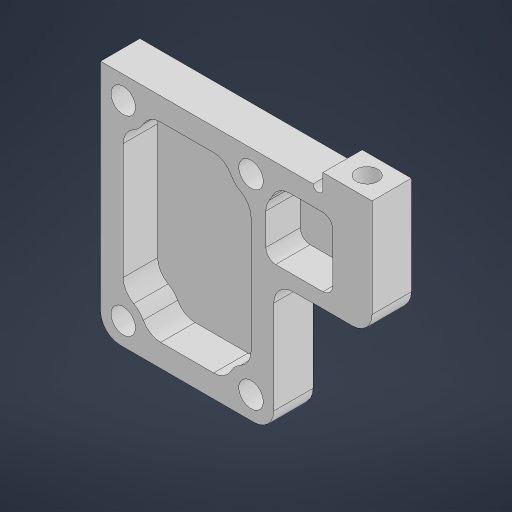
# Autodesk Inventor part: SolenoidMount
Saved by Autodesk Inventor 2024.2 (Build 282272000, 272)
## iProperties
Created: 2023-12-22
Part Number: SolenoidMount
Material: 一般
Document SubType Name: Modeling
Designer: Hanaoka
Density: 1 g/cm^3
Appearance: 既定
Author: Hanaoka
Autodesk Inventor part; units mm, degrees
ref_plane "YZ Plane" through (0, 0, 0) normal (1, 0, 0) x (0, 1, 0)
ref_plane "XZ Plane" through (0, 0, 0) normal (0, 1, 0) x (-1, 0, 0)
ref_plane "XY Plane" through (0, 0, 0) normal (0, 0, 1) x (1, 0, 0)
ref_plane "作業平面1" through (0, 0, 0.15) normal (0, 0, 1) x (1, 0, 0)
sketch "スケッチ1" plane through (0, 0, 0.15) normal (0, 0, 1) x (1, 0, 0)
  line L0 (0, -24) -> (-27.3, -24) projected
  line L1 (-3.7, -24) -> (-3.7, -10.5)
  line L2 (-3.7, -10.5) -> (4.3, -10.5)
  line L3 (6.3, -8.5) -> (6.3, 1.5)
  line L4 (6.3, 1.5) -> (1.3, 1.5)
  line L5 (-27.3, 0) -> (0, 0) projected
  line L6 (1.3, 1.5) -> (1.3, 0)
  circle A0 centre (-6, -21.7) radius 1.25 projected
  circle A1 centre (-19, -21.7) radius 1.25 projected
  circle A2 centre (-6, -21.7) radius 2.3 construction
  circle A3 centre (-19, -21.7) radius 2.3 construction
  line L7 (1.3, 0) -> (0, 0)
  line L8 (-21.3, -24) -> (-21.3, 0)
  circle A4 centre (-6, -2.3) radius 1.25 projected
  circle A5 centre (-19, -2.3) radius 1.25 projected
  line L9 (1.3, 0) -> (0.8, 0)
  arc A6 (0.3, 0) -> (1.3, 0) centre (0.8, 0) ccw
  line L10 (-6, -21.7) -> (-19, -21.7)
  line L11 (-19, -21.7) -> (-19, -2.3)
  line L12 (-19, -2.3) -> (-6, -2.3)
  line L13 (-6, -2.3) -> (-6, -21.7)
  arc A7 (-6, -19.4) -> (-8.3, -21.7) centre (-6, -21.7) ccw
  arc A8 (-16.7, -21.7) -> (-19, -19.4) centre (-19, -21.7) ccw
  arc A9 (-19, -4.6) -> (-16.7, -2.3) centre (-19, -2.3) ccw
  arc A10 (-8.3, -2.3) -> (-6, -4.6) centre (-6, -2.3) ccw
  arc A11 (4.3, -10.5) -> (6.3, -8.5) centre (4.3, -8.5) ccw
  line L14 (-3.5, -2) -> (1.3, -2)
  line L15 (2.3, -3) -> (2.3, -8)
  line L16 (1.3, -9) -> (-3.5, -9)
  line L17 (-4.5, -8) -> (-4.5, -3)
  arc A12 (1.3, -9) -> (2.3, -8) centre (1.3, -8) ccw
  arc A13 (2.3, -3) -> (1.3, -2) centre (1.3, -3) ccw
  arc A14 (-3.5, -2) -> (-4.5, -3) centre (-3.5, -3) ccw
  arc A15 (-4.5, -8) -> (-3.5, -9) centre (-3.5, -8) ccw
  arc A16 (-4.5, -4.0436) -> (-3.7196, -2) centre (-6, -2.3) ccw
  point P0 (6.3, -10.5)
  point P1 (0.8, -0.5)
  point P2 (-3.7167, -2.0238)
  dimension "d0" = 1.5
  dimension "d1" = 12
  dimension "d2" = 10
  dimension "d3" = 5
  dimension "d9" = 0.5
  dimension "d13" = 2
  dimension "d14" = 1
  dimension "d15" = 1.5
  dimension "d16" = 1.5
  dimension "d17" = 4
  dimension "d18" = 1.5
  constraints: 32 end point, 27 point on circle, 18 point on line, 14 tangent, 13 centre point, 8 coincident, 6 equal radius, 5 parallel, 4 horizontal, 3 vertical, 2 perpendicular, 1 collinear
  measures "d0" distance of L4.end L6.end
  measures "d1" distance of point (6.3, -10.5) L3.end
  measures "d2" distance of L1.end point (6.3, -10.5)
  measures "d3" distance of L3.end L4.end
  measures "d9" distance of L6.end L9.end
  measures "d13" radius of A11
  measures "d14" radius of A12
  measures "d15" distance between parallel lines of L2 L16
  measures "d16" distance from line of point (0.8, -0.5) L14
  measures "d17" distance between parallel lines of L3 L15
  measures "d18" distance between parallel lines of L13 L17
extrude "押し出し1" add sketch "スケッチ1" along normal blind 4 contours L0 L8 L5 L7 A6 L6 L4 L3 A11 L2 L1 | A0 L10 A7 L13 | A10 L12 A4 L13 | L10 A1 L11 A8 | A9 L11 A5 L12 | A16 L17 A14
sketch "スケッチ2" plane through (1.3, 1.5, 0.15) normal (0, 1, 0) x (1, 0, 0)
  line L0 (5, 0) -> (5, -4) projected
  line L1 (0, 0) -> (-22.6, 0) projected
  line L2 (5, -4) -> (0, 0) construction
  circle A0 centre (2.5, -2) radius 1.1
  point P0 (-1.3, 0.15)
  dimension "d6" = 2.2
  constraints: 2 end point, 1 centre point, 1 coincident, 1 midpoint, 1 other
  measures "d6" diameter of A0
extrude "押し出し2" cut sketch "スケッチ2" against normal blind 5
fillet "フィレット1" radius 2 13 edges at (-3.7, -10.5, 2.15) (-3.7, -24, 2.15) (-21.3, -24, 2.15) (-6, -19.4, 2.15) (-8.3, -21.7, 2.15) (-16.7, -21.7, 2.15) (-19, -19.4, 2.15) (-19, -4.6, 2.15) (-16.7, -2.3, 2.15) (-8.3, -2.3, 2.15) (-6, -4.6, 2.15) (-4.5, -4.0436, 2.15) (-3.7167, -2.0238, 2.15)
sketch "スケッチ3" plane through (0, 0, 0.15) normal (0, 0, -1) x (-1, 0, 0)
  arc A0 (19.3, -24) -> (21.3, -22) centre (19.3, -22) ccw projected
  line L0 (21.3, 0) -> (21.3, -22) projected
  line L1 (-0.3, 0) -> (21.3, 0) projected
  arc A1 (-1.3, 0) -> (-0.3, 0) centre (-0.8, 0) ccw projected
  line L2 (-1.3, 1.5) -> (-1.3, 0) projected
  line L3 (-6.3, 1.5) -> (-1.3, 1.5) projected
  line L4 (-6.3, -8.5) -> (-6.3, 1.5) projected
  arc A2 (-6.3, -8.5) -> (-4.3, -10.5) centre (-4.3, -8.5) ccw projected
  line L5 (1.7, -10.5) -> (-4.3, -10.5) projected
  arc A3 (3.7, -12.5) -> (1.7, -10.5) centre (1.7, -12.5) ccw projected
  line L6 (3.7, -22) -> (3.7, -12.5) projected
  arc A4 (3.7, -22) -> (5.7, -24) centre (5.7, -22) ccw projected
  line L7 (19.3, -24) -> (5.7, -24) projected
  circle A5 centre (6, -2.3) radius 1.25 projected
  arc A6 (9.8066, -2.3) -> (8.0361, -3.3698) centre (9.8066, -4.3) ccw projected
  line L8 (15.1934, -2.3) -> (9.8066, -2.3) projected
  arc A7 (16.9639, -3.3698) -> (15.1934, -2.3) centre (15.1934, -4.3) ccw projected
  arc A8 (16.9639, -3.3698) -> (17.9302, -4.3361) centre (19, -2.3) ccw projected
  arc A9 (19, -6.1066) -> (17.9302, -4.3361) centre (17, -6.1066) ccw projected
  line L9 (19, -17.8934) -> (19, -6.1066) projected
  arc A10 (17.9302, -19.6639) -> (19, -17.8934) centre (17, -17.8934) ccw projected
  arc A11 (17.9302, -19.6639) -> (16.9639, -20.6302) centre (19, -21.7) ccw projected
  arc A12 (15.1934, -21.7) -> (16.9639, -20.6302) centre (15.1934, -19.7) ccw projected
  line L10 (9.8066, -21.7) -> (15.1934, -21.7) projected
  arc A13 (8.0361, -20.6302) -> (9.8066, -21.7) centre (9.8066, -19.7) ccw projected
  arc A14 (8.0361, -20.6302) -> (7.0698, -19.6639) centre (6, -21.7) ccw projected
  arc A15 (6, -17.8934) -> (7.0698, -19.6639) centre (8, -17.8934) ccw projected
  line L11 (6, -6.1066) -> (6, -17.8934) projected
  arc A16 (7.0698, -4.3361) -> (6, -6.1066) centre (8, -6.1066) ccw projected
  arc A17 (7.0698, -4.3361) -> (8.0361, -3.3698) centre (6, -2.3) ccw projected
  circle A18 centre (19, -2.3) radius 1.25 projected
  circle A19 centre (19, -21.7) radius 1.25 projected
  line L12 (2.0503, -2) -> (-1.3, -2) projected
  arc A20 (3.8874, -3.2093) -> (4.1279, -3.6361) centre (6, -2.3) ccw projected
  line L13 (4.5, -8) -> (4.5, -4.798) projected
  arc A21 (3.5, -9) -> (4.5, -8) centre (3.5, -8) ccw projected
  line L14 (-1.3, -9) -> (3.5, -9) projected
  arc A22 (-2.3, -8) -> (-1.3, -9) centre (-1.3, -8) ccw projected
  line L15 (-2.3, -3) -> (-2.3, -8) projected
  arc A23 (-1.3, -2) -> (-2.3, -3) centre (-1.3, -3) ccw projected
  circle A24 centre (6, -21.7) radius 1.25 projected
  arc A25 (3.8874, -3.2093) -> (2.0503, -2) centre (2.0503, -4) ccw projected
  arc A26 (4.5, -4.798) -> (4.1279, -3.6361) centre (2.5, -4.798) ccw projected
  point P0 (0, 0)
extrude "押し出し3" add sketch "スケッチ3" against normal blind 0.5 contours L8 A7 A8 A9 L9 A10 A11 A12 L10 A13 A14 A15 L11 A16 A17 A6 | A25 A20 A26 L13 A21 L14 A22 L15 A23 L12
